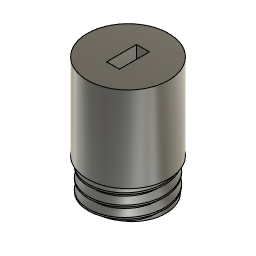
Threaded Breadboard Peg (Autodesk Fusion 360 design; units mm, degrees)
Autodesk Fusion 360 part; units mm, degrees
sketch "Sketch1" plane through (0, 0, 0) normal (0, 0, 1) x (1, 0, 0) in component "Breadboard Peg"
  circle A0 centre (0, 0) radius 4.75
  dimension "d1" = 9.5
  constraint coincident A0.centre origin
  measures "d1" diameter of A0
extrude "Extrude1" add sketch "Sketch1" along normal blind 20 in component "Breadboard Peg"
sketch "Sketch1 (2)" plane through (0, 0, 0) normal (0, 0, -1) x (1, 0, 0)
  circle A0 centre (0, 0) radius 4.75
  circle A1 centre (0, 0) radius 4.5
  dimension "d4" = 9
  constraint coincident A0.centre A1.centre
  measures "d4" diameter of A1
extrude "Extrude2" cut sketch "Sketch1 (2)" against normal blind 10 in component "Breadboard Peg"
sketch "Sketch2" plane through (0, 0, 20) normal (0, 0, 1) x (-1, 0, 0)
  circle A0 centre (0, 0) radius 4.75
  line L0 (-0.75, -1.75) -> (0.75, -1.75)
  line L1 (0.75, -1.75) -> (0.75, 1.75)
  line L2 (0.75, 1.75) -> (-0.75, 1.75)
  line L3 (-0.75, 1.75) -> (-0.75, -1.75)
  line L4 (-0.75, -1.75) -> (0.75, 1.75) construction
  line L5 (0.75, -1.75) -> (-0.75, 1.75) construction
  dimension "d7" = 1.5
  dimension "d8" = 3.5
  constraint horizontal L0
  constraint perpendicular L0 L1
  constraint parallel L0 L2
  constraint parallel L1 L3
  constraint coincident L4 A0.centre
  constraint coincident L5 A0.centre
  constraint coincident A0.centre origin
  measures "d7" distance of L1.end L2.end
  measures "d8" distance of L0.end L1.end
extrude "Extrude3" cut sketch "Sketch2" against normal blind 3.5 contours L0 L1 L2 L3 in component "Breadboard Peg"
extrude "Extrude4" cut 1 faces at (-0.0731, 0.976, 0) along direction (0, 0, 1) blind 6 in component "Breadboard Peg"
thread "Thread2" "ISO Metric profile 9.0 M9x1.25 6g" major diameter 8.866 minor diameter 7.4455 pitch 1.25 angle 60 modelled right hand crest width 0.1834 on face at (4.4776, 0.4481, 7.3333) crest through (4.433, 0, 5.6875) in component "Breadboard Peg"
component "Breadboard Peg" placed x (1, 0, 0) y (0, 1, 0) z (0, 0, 1) at (0, 0, 0)
named bodies: "Breadboard Peg"
